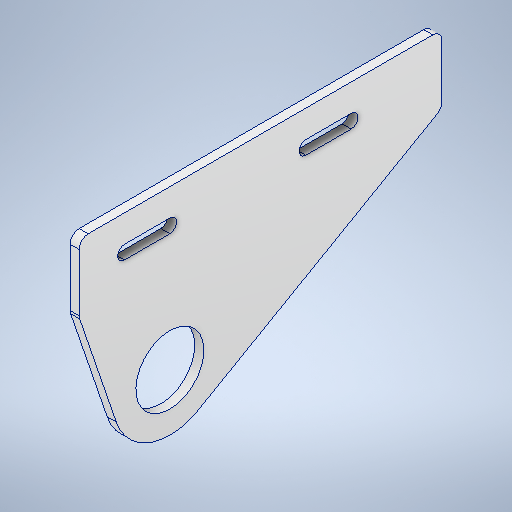
# Autodesk Inventor part: ball_loading_v1_Plate_up_F
Saved by Autodesk Inventor 2025.1 (Build 291241000, 241)
## iProperties
Created: 2024-11-12
Part Number: ball_loading_v1_Plate_up_F
Material: アルミニウム 6061
Document SubType Name: Modeling
Designer: haruy
Density: 2.7 g/cm^3
Appearance: アルミニウム - フラット
Author: haruy
Autodesk Inventor part; units mm, degrees
ref_plane "YZ Plane" through (0, 0, 0) normal (1, 0, 0) x (0, 1, 0)
ref_plane "XZ Plane" through (0, 0, 0) normal (0, 1, 0) x (-1, 0, 0)
ref_plane "XY Plane" through (0, 0, 0) normal (0, 0, 1) x (1, 0, 0)
derived "ball_loading_v1_Sketch_Base.ipt"
sketch "スケッチ3" plane through (200, 0, 0) normal (1, 0, 0) x (0, 1, 0)
  line L0 (0, 0) -> (305, 0)
  line L1 (305, 0) -> (305, -15)
  line L2 (305, -15) -> (0, -15)
  line L3 (0, -15) -> (0, 0)
  line L4 (0, 35) -> (-15, 35)
  line L5 (-15, 35) -> (-15, -192.5)
  line L6 (-15, -192.5) -> (0, -192.5)
  line L7 (0, -192.5) -> (0, 35)
  line L8 (0, 35) -> (-15, 35)
  line L9 (-15, 35) -> (-15, 20)
  line L10 (-15, 20) -> (0, 20)
  line L11 (0, 20) -> (0, 35)
  line L12 (50, -15) -> (65, -15)
  line L13 (65, -15) -> (65, -192.5)
  line L14 (65, -192.5) -> (50, -192.5)
  line L15 (50, -192.5) -> (50, -15)
  line L16 (305, -15) -> (290, -15)
  line L17 (290, -15) -> (290, -192.5)
  line L18 (290, -192.5) -> (305, -192.5)
  line L19 (305, -192.5) -> (305, -15)
  circle A0 centre (25, -60) radius 12.5
  circle A1 centre (25, -100) radius 18.75
  line L20 (305, -192.5) -> (0, -192.5)
  line L21 (-15, -40) -> (65, -40)
  line L22 (65, -120) -> (-15, -120)
  circle A2 centre (25, -100) radius 20
  line L23 (42.5, 0) -> (42.5, -15)
  line L24 (65, -15) -> (65, 0)
  line L25 (20, 0) -> (20, -15)
  line L26 (0, 7.5) -> (-15, 7.5)
  line L27 (0, -22.5) -> (-15, -22.5)
  circle A3 centre (270, -60) radius 12.5
  line L28 (305, -35) -> (290, -35)
  line L29 (282.5, 0) -> (282.5, -15)
  line L30 (0, -385) -> (305, -385)
  line L31 (305, -370) -> (0, -370)
  line L32 (0, -370) -> (0, -385)
  circle A4 centre (25, -325) radius 12.5
  line L33 (-15, -345) -> (65, -345)
  line L34 (0, -362.5) -> (-15, -362.5)
  line L35 (50, -370) -> (65, -370)
  line L36 (65, -370) -> (65, -385)
  line L37 (42.5, -385) -> (42.5, -370)
  line L38 (20, -385) -> (20, -370)
  line L39 (65, -265) -> (-15, -265)
  circle A5 centre (25, -285) radius 18.75
  circle A6 centre (25, -285) radius 20
  line L40 (65, -370) -> (65, -192.5)
  line L41 (50, -192.5) -> (50, -370)
  line L42 (0, -192.5) -> (0, -420)
  line L43 (-15, -420) -> (-15, -192.5)
  line L44 (0, -420) -> (-15, -420)
  line L45 (282.5, -385) -> (282.5, -370)
  line L46 (305, -370) -> (290, -370)
  line L47 (305, -385) -> (305, -370)
  line L48 (305, -350) -> (290, -350)
  line L49 (290, -370) -> (290, -192.5)
  line L50 (305, -192.5) -> (305, -370)
  circle A7 centre (270, -325) radius 12.5
  line L51 (0, -420) -> (-15, -420)
  line L52 (-15, -420) -> (-15, -405)
  line L53 (-15, -405) -> (0, -405)
  line L54 (0, -405) -> (0, -420)
  line L55 (0, -392.5) -> (-15, -392.5)
  line L56 (305, -40) -> (257.5, -40)
  line L57 (257.5, -40) -> (257.5, -120)
  line L58 (257.5, -120) -> (305, -120)
  line L59 (305, -120) -> (305, -40)
  line L60 (290, -40) -> (265.9774, -48.1649)
  line L61 (259.1566, -66.2186) -> (290, -120)
  circle A8 centre (270, -60) radius 7.5
  circle A9 centre (297.5, -60) radius 1.5
  circle A10 centre (297.5, -100) radius 1.5
  circle A11 centre (297.5, -90) radius 1.5
  circle A12 centre (297.5, -50) radius 1.5
  line L62 (299, -50) -> (299, -60)
  line L63 (296, -50) -> (296, -60)
  line L64 (299, -90) -> (299, -100)
  line L65 (296, -90) -> (296, -100)
  point P0 (290, -103.75)
  point P1 (305, -120)
  dimension "d1" = 15
  dimension "d2" = 3
  dimension "d3" = 3
  dimension "d4" = 3
  dimension "d5" = 3
  dimension "d6" = 10
  dimension "d7" = 7.5
  dimension "d8" = 7.5
  dimension "d9" = 10
  measures "d1" diameter of A8
  measures "d2" diameter of A9
  measures "d3" diameter of A10
  measures "d4" diameter of A11
  measures "d5" diameter of A12
  measures "d6" distance of A9.centre A12.centre
  measures "d7" distance from line of L19 A12.centre
  measures "d8" distance from line of L19 A11.centre
  measures "d9" distance of A10.centre A11.centre
ref_plane "作業平面1" through (200, 0, 0) normal (1, 0, 0) x (0, 1, 0)
ref_plane "作業平面2" through (0, 0, 200) normal (0, 0, 1) x (1, 0, 0)
extrude "押し出し1" add sketch "スケッチ3" along normal blind 2 contours L19 L58 L17 L56 | L17 L61 A3 L60 | A3
fillet "フィレット1" radius 2 4 edges at (201, 305, -40) (201, 290, -40) (201, 305, -120) (201, 290, -120)
sketch "スケッチ4" plane through (202, 290.3306, -40) normal (1, 0, 0) x (0, 0, -1)
  arc A0 (78.995, -0.907) -> (80, 0.828) centre (78, 0.828) ccw projected
  line L0 (80, 0.828) -> (80, 12.6694) projected
  arc A1 (80, 12.6694) -> (78, 14.6694) centre (78, 12.6694) ccw projected
  line L1 (78, 14.6694) -> (2, 14.6694) projected
  arc A2 (2, 14.6694) -> (0, 12.6694) centre (2, 12.6694) ccw projected
  line L2 (0, 12.6694) -> (0, 0) projected
  arc A3 (0, 0) -> (0.1064, -0.6436) centre (2, 0) ccw projected
  line L3 (0.1064, -0.6436) -> (8.1649, -24.3532) projected
  arc A4 (8.1649, -24.3532) -> (26.2186, -31.174) centre (20, -20.3306) ccw projected
  line L4 (26.2186, -31.174) -> (78.995, -0.907) projected
  circle A5 centre (20, -20.3306) radius 7.5 projected
  line L5 (10, 8.6694) -> (20, 8.6694) projected
  arc A6 (20, 5.6694) -> (20, 8.6694) centre (20, 7.1694) ccw projected
  line L6 (20, 5.6694) -> (10, 5.6694) projected
  arc A7 (10, 8.6694) -> (10, 5.6694) centre (10, 7.1694) ccw projected
  line L7 (50, 8.6694) -> (60, 8.6694) projected
  arc A8 (60, 5.6694) -> (60, 8.6694) centre (60, 7.1694) ccw projected
  line L8 (60, 5.6694) -> (50, 5.6694) projected
  arc A9 (50, 8.6694) -> (50, 5.6694) centre (50, 7.1694) ccw projected
  point P0 (-40, -290.3306)
sketch "スケッチ2" plane through (0, 0, 200) normal (0, 0, 1) x (1, 0, 0)
  line L0 (0, 0) -> (-15, 0) projected
  line L1 (-15, 0) -> (-15, 248.5284) projected
  line L2 (-15, 248.5284) -> (0, 248.5284) projected
  line L3 (0, 248.5284) -> (0, 0) projected
  line L4 (-320, 0) -> (-305, 0) projected
  line L5 (-305, 0) -> (-305, 238.0267) projected
  line L6 (-305, 238.0267) -> (-320, 238.0267) projected
  line L7 (-320, 238.0267) -> (-320, 0) projected
  line L8 (-320, 0) -> (-324, 0) projected
  line L9 (-324, 0) -> (-324, 76.8713) projected
  line L10 (-324, 76.8713) -> (-320, 76.8713) projected
  line L11 (-320, 76.8713) -> (-320, 0) projected
  line L12 (-15, 0) -> (-19, 0) projected
  line L13 (-19, 0) -> (-19, 51.1976) projected
  line L14 (-19, 51.1976) -> (-15, 51.1976) projected
  line L15 (-15, 51.1976) -> (-15, 0) projected
  line L16 (-335, 13.6956) -> (-4, 13.6956) projected
  line L17 (-4, 13.6956) -> (-4, 23.6956) projected
  line L18 (-4, 23.6956) -> (-335, 23.6956) projected
  line L19 (-335, 23.6956) -> (-335, 13.6956) projected
  line L20 (-216, 31.1956) -> (-114, 31.1956) projected
  line L21 (-114, 31.1956) -> (-114, 6.1956) projected
  line L22 (-114, 6.1956) -> (-216, 6.1956) projected
  line L23 (-216, 6.1956) -> (-216, 31.1956) projected
  line L24 (-150, 31.1956) -> (-146, 31.1956) projected
  line L25 (-146, 31.1956) -> (-146, 6.1956) projected
  line L26 (-146, 6.1956) -> (-150, 6.1956) projected
  line L27 (-150, 6.1956) -> (-150, 31.1956) projected
  line L28 (-198, 31.1956) -> (-194, 31.1956) projected
  line L29 (-194, 31.1956) -> (-194, 6.1956) projected
  line L30 (-194, 6.1956) -> (-198, 6.1956) projected
  line L31 (-198, 6.1956) -> (-198, 31.1956) projected
  line L32 (-126, 31.1956) -> (-122, 31.1956) projected
  line L33 (-122, 31.1956) -> (-122, 6.1956) projected
  line L34 (-122, 6.1956) -> (-126, 6.1956) projected
  line L35 (-126, 6.1956) -> (-126, 31.1956) projected
  circle A0 centre (-165.0738, 76.8713) radius 120 projected
  line L36 (-174, 31.1956) -> (-170, 31.1956) projected
  line L37 (-170, 31.1956) -> (-170, 6.1956) projected
  line L38 (-170, 6.1956) -> (-174, 6.1956) projected
  line L39 (-174, 6.1956) -> (-174, 31.1956) projected
  line L40 (-160, 31.1956) -> (-160, 6.1956) projected
